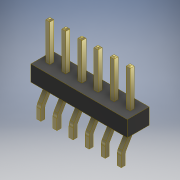
# Autodesk Inventor part: SMD2.54-1x06-R
Saved by Autodesk Inventor 2018 (Build 220112000, 112)
## iProperties
Created: 2018-06-05
Part Number: SMD2.54-1x06-R
Material: Nickel-Copper Alloy 400
Document SubType Name: Modeling
Designer: Bradley
Density: 8.83 g/cm^3
Appearance: Gold - Metal
Author: Bradley
Autodesk Inventor part; units mm, degrees
ref_plane "YZ Plane" through (0, 0, 0) normal (1, 0, 0) x (0, 1, 0)
ref_plane "XZ Plane" through (0, 0, 0) normal (0, 1, 0) x (-1, 0, 0)
ref_plane "XY Plane" through (0, 0, 0) normal (0, 0, 1) x (1, 0, 0)
sketch "Sketch1" plane through (0, 0, 0) normal (1, 0, 0) x (0, 1, 0)
  line L0 (2.05, 7.24) -> (2.05, -1.3)
  arc A0 (1.8703, -1.9539) -> (2.05, -1.3) centre (0.77, -1.3) ccw
  line L1 (1.8703, -1.9539) -> (0.7298, -3.873)
  arc A1 (0.7298, -3.873) -> (0.64, -4.2) centre (1.28, -4.2) ccw
  line L2 (0.64, -4.2) -> (0.64, -6)
  line L3 (0.64, -6) -> (0, -6)
  line L4 (0, -6) -> (0, -4.2)
  arc A2 (0.1797, -3.5461) -> (0, -4.2) centre (1.28, -4.2) ccw
  line L5 (0.1797, -3.5461) -> (1.3202, -1.627)
  arc A3 (1.3202, -1.627) -> (1.41, -1.3) centre (0.77, -1.3) ccw
  line L6 (1.41, -1.3) -> (1.41, 7.24)
  line L7 (1.41, 7.24) -> (2.05, 7.24)
  point P0 (0, 0)
  dimension "d0" = 0.64
  dimension "d1" = 13.24
  dimension "d2" = 1.8
  dimension "d3" = 4.7
  dimension "d4" = 1.41
  dimension "d5" = 0.64
  dimension "d6" = 6
  constraints: 16 end point, 8 point on circle, 7 tangent, 4 centre point, 3 parallel, 3 perpendicular, 2 concentric, 2 equal radius, 1 point on line, 1 vertical
  measures "d0" distance of L2.end L3.end
  measures "d1" distance between parallel lines of L7 L3
  measures "d2" distance from line of A1.centre L3
  measures "d3" distance from line of A0.centre L3
  measures "d4" distance between parallel lines of L4 L6
  measures "d5" radius of A1
  measures "d6" distance from line of point (0, 0) L3
extrude "Extrusion1" add sketch "Sketch1" along normal mid plane 0.64
chamfer "Chamfer1" distance 0.175 angle 45 8 edges at (0, 2.05, 7.24) (-0.32, 1.73, 7.24) (0, 1.41, 7.24) (0.32, 1.73, 7.24) (0, 0.64, -6) (-0.32, 0.32, -6) (0, 0, -6) (0.32, 0.32, -6)
pattern_linear "Rectangular Pattern1" count 6 spacing 2.54 along (1, 0, 0) of "Extrusion1", "Chamfer1"
sketch "Sketch2" plane through (0, 0, 0) normal (0, 0, 1) x (1, 0, 0)
  line L0 (-1.27, 3.46) -> (13.97, 3.46)
  line L1 (13.97, 3.46) -> (13.97, 0)
  line L2 (13.97, 0) -> (-1.27, 0)
  line L3 (-1.27, 0) -> (-1.27, 3.46)
  line L4 (0.32, 1.41) -> (-0.32, 1.41) projected
  line L5 (0.32, 2.05) -> (0.32, 1.41) projected
  line L6 (-0.32, 2.05) -> (0.32, 2.05) projected
  line L7 (-0.32, 1.41) -> (-0.32, 2.05) projected
  line L8 (13.02, 1.41) -> (12.38, 1.41) projected
  line L9 (13.02, 2.05) -> (13.02, 1.41) projected
  line L10 (12.38, 2.05) -> (13.02, 2.05) projected
  line L11 (12.38, 1.41) -> (12.38, 2.05) projected
  line L12 (12.38, 1.73) -> (0.32, 1.73) construction
  point P0 (0, 0)
  point P1 (6.35, 1.73)
  point P2 (6.35, 3.46)
  dimension "d12" = 3.46
  dimension "d13" = 15.24
  constraints: 10 end point, 4 midpoint, 2 parallel, 2 perpendicular, 1 horizontal, 1 point on line, 1 vertical alignment
  measures "d12" distance of L2.end L0.start
  measures "d13" distance of L1.end L2.end
extrude "Extrusion2" add sketch "Sketch2" along normal mid plane 2.5
equation "\"d7\" = d0"
body "Solid1"
